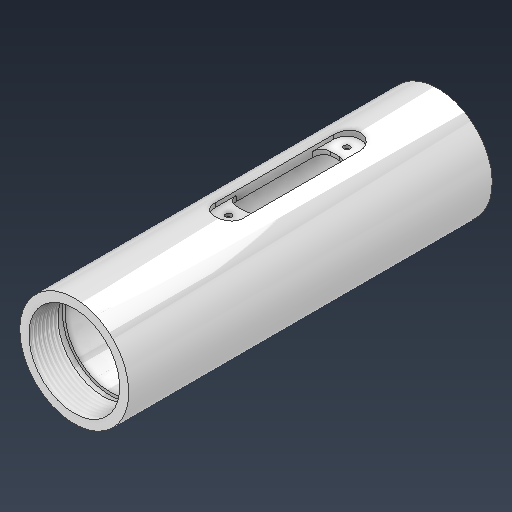
# Autodesk Inventor part: InventorNativeNewHilt
Saved by Autodesk Inventor 2025.1 (Build 291241000, 241)
## iProperties
Created: 2024-08-20
Part Number: InventorNativeNewHilt
Material: Aluminum 6061
Document SubType Name: Modeling
Designer: Michael
Density: 2.7 g/cm^3
Appearance: Aluminum - Polished
Mass: 114.553 g
Surface Area: 287.051 cm^2
Volume: 42.427 cm^3
Author: Michael
Autodesk Inventor part; units mm, degrees
ref_plane "YZ Plane" through (0, 0, 0) normal (1, 0, 0) x (0, 1, 0)
ref_plane "XY Plane" through (0, 0, 0) normal (0, 0, 1) x (1, 0, 0)
sketch "Sketch1" plane through (0, 0, 0) normal (0, 0, 1) x (1, 0, 0)
  line L0 (-106.628, 0) -> (106.628, 0) construction
  line L1 (-63.5, 19.05) -> (63.5, 19.05)
  line L2 (63.5, 19.05) -> (63.5, 15.875)
  line L3 (-63.5, 15.875) -> (-63.5, 19.05)
  line L4 (-63.5, 15.875) -> (-53.34, 15.875)
  line L5 (-53.34, 15.875) -> (-53.34, 16.891)
  line L6 (-53.34, 16.891) -> (-50.8, 16.891)
  line L7 (-50.8, 16.891) -> (-50.8, 15.875)
  line L8 (-50.8, 15.875) -> (0, 15.875)
  line L9 (0, 0) -> (0, 19.05) construction
  line L10 (63.5, 15.875) -> (53.34, 15.875)
  line L11 (53.34, 15.875) -> (53.34, 16.891)
  line L12 (53.34, 16.891) -> (50.8, 16.891)
  line L13 (50.8, 16.891) -> (50.8, 15.875)
  line L14 (50.8, 15.875) -> (0, 15.875)
  dimension "d0" = 127
  dimension "d1" = 38.1
  dimension "d2" = 31.75
  dimension "d3" = 10.16
  dimension "d4" = 2.54
  dimension "d5" = 1.016
  constraints: 30 end point, 4 perpendicular, 4 point on line, 4 symmetric about line, 3 horizontal, 2 midpoint, 1 coincident, 1 horizontal alignment, 1 parallel, 1 vertical, 1 vertical alignment
  measures "d0" distance between parallel lines of L2 L3
  measures "d1" diameter of L1 L0
  measures "d2" diameter of L8 L0
  measures "d3" distance between parallel lines of L3 L5
  measures "d4" distance of L5.end L6.end
  measures "d5" distance between parallel lines of L6 L4
revolve "Revolution1" add sketch "Sketch1" angle 360 about axis through (-106.628, 0, 0) along (1, 0, 0)
ref_plane "Work Plane1" through (0, 19.05, 0) normal (0, 1, 0) x (-1, 0, 0)
sketch "Sketch2" plane through (0, 19.05, 0) normal (0, 1, 0) x (-1, 0, 0)
  line L0 (-31.75, 0) -> (9.525, 0) construction
  line L1 (-31.75, -4.7625) -> (9.525, -4.7625)
  line L2 (9.525, 4.7625) -> (-31.75, 4.7625)
  arc A0 (-31.75, 4.7625) -> (-31.75, -4.7625) centre (-31.75, 0) ccw
  arc A1 (9.525, -4.7625) -> (9.525, 4.7625) centre (9.525, 0) ccw
  line L3 (-63.5, 19.05) -> (-63.5, -19.05) projected
  line L4 (-27.6225, 1.5875) -> (-27.6225, -1.5875)
  line L5 (5.3975, 1.5875) -> (5.3975, -1.5875)
  arc A2 (5.3975, 1.5875) -> (2.2225, 4.7625) centre (2.2225, 1.5875) ccw
  arc A3 (2.2225, -4.7625) -> (5.3975, -1.5875) centre (2.2225, -1.5875) ccw
  arc A4 (-24.4475, 4.7625) -> (-27.6225, 1.5875) centre (-24.4475, 1.5875) ccw
  arc A5 (-27.6225, -1.5875) -> (-24.4475, -4.7625) centre (-24.4475, -1.5875) ccw
  point P0 (0, 0)
  point P1 (-11.1125, 0)
  point P2 (-36.5125, 0)
  point P3 (9.525, 0)
  point P4 (-63.5, 0)
  dimension "d7" = 9.525
  dimension "d8" = 41.275
  dimension "d10" = 33.02
  dimension "d11" = 16.51
  dimension "d12" = 3.175
  dimension "d13" = 3.175
  dimension "d27" = 31.75
  constraints: 13 point on circle, 12 end point, 12 tangent, 6 centre point, 4 point on line, 2 coincident, 2 midpoint, 2 perpendicular, 1 equal radius, 1 horizontal, 1 horizontal alignment, 1 parallel, 1 vertical alignment
  measures "d7" distance between parallel lines of L2 L1
  measures "d8" distance of L0.start L0.end
  measures "d10" distance between parallel lines of L4 L5
  measures "d11" distance from line of L5 point (-11.112, 0)
  measures "d12" radius of A2
  measures "d13" radius of A4
  measures "d27" distance of point (-63.5, 0) point (-31.75, 0)
extrude "Extrusion1" cut sketch "Sketch2" against normal blind 2.032
extrude "Extrusion2" cut sketch "Sketch2" against normal up to surface contours A5 L4 A4 L2 A2 L5 A3 L1
hole "Hole1" at (-9.525, 19.05, 0) at (31.75, 19.05, 0) direction (0, -1, 0) diameter 2.1565 depth 6.35 tip angle 118 thread size "4-40 UNC" class "2B" standard "ANSI Unified Screw Threads"
thread "Thread1" size "1 1/4-18 UNEF" class "2B" standard "ANSI Unified Screw Threads" full length
equation "\"d11\" = 0.5 * d10"
